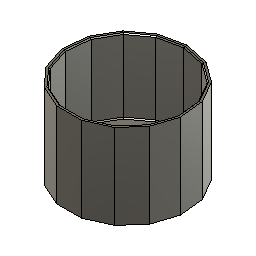
BraunBowl (Autodesk Fusion 360 design; units mm, degrees)
Autodesk Fusion 360 part; units mm, degrees
sketch "Sketch1" plane through (0, 0, 0) normal (0, 1, 0) x (1, 0, 0)
  line L0 (0, 59) -> (-23.9975, 53.8992)
  line L1 (-23.9975, 53.8992) -> (-43.8455, 39.4787)
  line L2 (-43.8455, 39.4787) -> (-56.1123, 18.232)
  line L3 (-56.1123, 18.232) -> (-58.6768, -6.1672)
  line L4 (-58.6768, -6.1672) -> (-51.0955, -29.5)
  line L5 (-51.0955, -29.5) -> (-34.6793, -47.732)
  line L6 (-34.6793, -47.732) -> (-12.2668, -57.7107)
  line L7 (-12.2668, -57.7107) -> (12.2668, -57.7107)
  line L8 (12.2668, -57.7107) -> (34.6793, -47.732)
  line L9 (34.6793, -47.732) -> (51.0955, -29.5)
  line L10 (51.0955, -29.5) -> (58.6768, -6.1672)
  line L11 (58.6768, -6.1672) -> (56.1123, 18.232)
  line L12 (56.1123, 18.232) -> (43.8455, 39.4787)
  line L13 (43.8455, 39.4787) -> (23.9975, 53.8992)
  line L14 (23.9975, 53.8992) -> (0, 59)
extrude "Extrude1" add sketch "Sketch1" along normal blind 84
sketch "Sketch2" plane through (0, 84, 0) normal (0, 1, 0) x (-1, 0, 0)
  line L0 (0, -56) -> (22.7773, -51.1585)
  line L1 (22.7773, -51.1585) -> (41.6161, -37.4713)
  line L2 (41.6161, -37.4713) -> (53.2592, -17.305)
  line L3 (53.2592, -17.305) -> (55.6932, 5.8536)
  line L4 (55.6932, 5.8536) -> (48.4974, 28)
  line L5 (48.4974, 28) -> (32.916, 45.305)
  line L6 (32.916, 45.305) -> (11.6431, 54.7763)
  line L7 (11.6431, 54.7763) -> (-11.6431, 54.7763)
  line L8 (-11.6431, 54.7763) -> (-32.916, 45.305)
  line L9 (-32.916, 45.305) -> (-48.4974, 28)
  line L10 (-48.4974, 28) -> (-55.6932, 5.8536)
  line L11 (-55.6932, 5.8536) -> (-53.2592, -17.305)
  line L12 (-53.2592, -17.305) -> (-41.6161, -37.4713)
  line L13 (-41.6161, -37.4713) -> (-22.7773, -51.1585)
  line L14 (-22.7773, -51.1585) -> (0, -56)
  line L15 (-23.9975, -53.8992) -> (0, -59)
  line L16 (0, -59) -> (23.9975, -53.8992)
  line L17 (23.9975, -53.8992) -> (43.8455, -39.4787)
  line L18 (43.8455, -39.4787) -> (56.1123, -18.232)
  line L19 (56.1123, -18.232) -> (58.6768, 6.1672)
  line L20 (58.6768, 6.1672) -> (51.0955, 29.5)
  line L21 (51.0955, 29.5) -> (34.6793, 47.732)
  line L22 (34.6793, 47.732) -> (12.2668, 57.7107)
  line L23 (12.2668, 57.7107) -> (-12.2668, 57.7107)
  line L24 (-12.2668, 57.7107) -> (-34.6793, 47.732)
  line L25 (-34.6793, 47.732) -> (-51.0955, 29.5)
  line L26 (-51.0955, 29.5) -> (-58.6768, 6.1672)
  line L27 (-58.6768, 6.1672) -> (-56.1123, -18.232)
  line L28 (-56.1123, -18.232) -> (-43.8455, -39.4787)
  line L29 (-43.8455, -39.4787) -> (-23.9975, -53.8992)
  dimension "d4" = 56
  measures "d4" distance of L0.start origin
extrude "Extrude2" cut sketch "Sketch2" against normal blind 72.8 contours L0 L1 L2 L3 L4 L5 L6 L7 L8 L9 L10 L11 L12 L13 L14
sketch "Sketch3" plane through (0, 11.2, 0) normal (0, 1, 0) x (-1, 0, 0)
  line L0 (-22.7773, -51.1585) -> (0, -56)
  line L1 (0, -56) -> (22.7773, -51.1585)
  line L2 (22.7773, -51.1585) -> (41.6161, -37.4713)
  line L3 (41.6161, -37.4713) -> (53.2592, -17.305)
  line L4 (53.2592, -17.305) -> (55.6932, 5.8536)
  line L5 (55.6932, 5.8536) -> (48.4974, 28)
  line L6 (48.4974, 28) -> (32.916, 45.305)
  line L7 (32.916, 45.305) -> (11.6431, 54.7763)
  line L8 (11.6431, 54.7763) -> (-11.6431, 54.7763)
  line L9 (-11.6431, 54.7763) -> (-32.916, 45.305)
  line L10 (-32.916, 45.305) -> (-48.4974, 28)
  line L11 (-48.4974, 28) -> (-55.6932, 5.8536)
  line L12 (-55.6932, 5.8536) -> (-53.2592, -17.305)
  line L13 (-53.2592, -17.305) -> (-41.6161, -37.4713)
  line L14 (-41.6161, -37.4713) -> (-22.7773, -51.1585)
  circle A0 centre (0, 0) radius 7.5
  dimension "d7" = 15
  constraint coincident A0.centre origin
  measures "d7" diameter of A0
extrude "Extrude3" add sketch "Sketch3" along normal blind 8 contours A0
chamfer "Chamfer1" distance 8 angle 45 1 edges at (6.9925, 11.2, 2.7121)
sketch "Sketch4" plane through (0, 19.2, 0) normal (0, 1, 0) x (-1, 0, 0)
  circle A0 centre (0, 0) radius 7.5
  circle A1 centre (0, 0) radius 3.9
  dimension "d11" = 7.8
  constraint coincident A0.centre A1.centre
  measures "d11" diameter of A1
extrude "Extrude4" cut sketch "Sketch4" against normal blind 14 contours A1
chamfer "Chamfer2" distance 1 angle 45 15 edges at (54.4762, 84, -5.7257) (47.4376, 84, -27.3881) (32.1967, 84, -44.3149) (-11.3886, 84, -53.5793) (11.3886, 84, -53.5793) (-32.1967, 84, -44.3149) (-47.4376, 84, -27.3881) (-54.4762, 84, -5.7257) (-52.0953, 84, 16.9268) (-40.7067, 84, 36.6525) (-22.2795, 84, 50.0406) (0, 84, 54.7763) (22.2795, 84, 50.0406) (40.7067, 84, 36.6525) (52.0953, 84, 16.9268)
chamfer "Chamfer4" distance 1 angle 45 3 edges at (-11.3886, 11.2, -53.5793) (11.3886, 11.2, -53.5793) (32.1967, 11.2, -44.3149) 1 faces at (-35.8936, 11.2, -21.1689)
sketch "Sketch7" plane through (0, 0, 0) normal (0, -1, 0) x (1, 0, 0)
  line L0 (0, -59) -> (23.9975, -53.8992)
  line L1 (23.9975, -53.8992) -> (43.8455, -39.4787)
  line L2 (43.8455, -39.4787) -> (56.1123, -18.232)
  line L3 (56.1123, -18.232) -> (58.6768, 6.1672)
  line L4 (58.6768, 6.1672) -> (51.0955, 29.5)
  line L5 (51.0955, 29.5) -> (34.6793, 47.732)
  line L6 (34.6793, 47.732) -> (12.2668, 57.7107)
  line L7 (12.2668, 57.7107) -> (-12.2668, 57.7107)
  line L8 (-12.2668, 57.7107) -> (-34.6793, 47.732)
  line L9 (-34.6793, 47.732) -> (-51.0955, 29.5)
  line L10 (-51.0955, 29.5) -> (-58.6768, 6.1672)
  line L11 (-58.6768, 6.1672) -> (-56.1123, -18.232)
  line L12 (-56.1123, -18.232) -> (-43.8455, -39.4787)
  line L13 (-43.8455, -39.4787) -> (-23.9975, -53.8992)
  line L14 (-23.9975, -53.8992) -> (0, -59)
  line L15 (0, -51.6115) -> (19.7509, -47.6828)
  line L16 (19.7509, -47.6828) -> (36.4949, -36.4949)
  line L17 (36.4949, -36.4949) -> (47.6828, -19.7509)
  line L18 (47.6828, -19.7509) -> (51.6115, 0)
  line L19 (51.6115, 0) -> (47.6828, 19.7509)
  line L20 (47.6828, 19.7509) -> (36.4949, 36.4949)
  line L21 (36.4949, 36.4949) -> (19.7509, 47.6828)
  line L22 (19.7509, 47.6828) -> (0, 51.6115)
  line L23 (0, 51.6115) -> (-19.7509, 47.6828)
  line L24 (-19.7509, 47.6828) -> (-36.4949, 36.4949)
  line L25 (-36.4949, 36.4949) -> (-47.6828, 19.7509)
  line L26 (-47.6828, 19.7509) -> (-51.6115, 0)
  line L27 (-51.6115, 0) -> (-47.6828, -19.7509)
  line L28 (-47.6828, -19.7509) -> (-36.4949, -36.4949)
  line L29 (-36.4949, -36.4949) -> (-19.7509, -47.6828)
  line L30 (-19.7509, -47.6828) -> (0, -51.6115)
  line L31 (-0.8802, -19.9806) -> (6.8331, -18.7965)
  line L32 (6.8331, -18.7965) -> (13.506, -14.7508)
  line L33 (13.506, -14.7508) -> (18.1228, -8.4595)
  line L34 (18.1228, -8.4595) -> (19.9806, -0.8802)
  line L35 (19.9806, -0.8802) -> (18.7965, 6.8331)
  line L36 (18.7965, 6.8331) -> (14.7508, 13.506)
  line L37 (14.7508, 13.506) -> (8.4595, 18.1228)
  line L38 (8.4595, 18.1228) -> (0.8802, 19.9806)
  line L39 (0.8802, 19.9806) -> (-6.8331, 18.7965)
  line L40 (-6.8331, 18.7965) -> (-13.506, 14.7508)
  line L41 (-13.506, 14.7508) -> (-18.1228, 8.4595)
  line L42 (-18.1228, 8.4595) -> (-19.9806, 0.8802)
  line L43 (-19.9806, 0.8802) -> (-18.7965, -6.8331)
  line L44 (-18.7965, -6.8331) -> (-14.7508, -13.506)
  line L45 (-14.7508, -13.506) -> (-8.4595, -18.1228)
  line L46 (-8.4595, -18.1228) -> (-0.8802, -19.9806)
  dimension "d29" = 20
  measures "d29" distance of L31.start origin
extrude "Extrude9" cut sketch "Sketch7" against normal blind 10 contours L15 L16 L17 L18 L19 L20 L21 L22 L23 L24 L25 L26 L27 L28 L29 L30
extrude "Extrude10" add 1 faces at (-21.5684, 10, -34.1002) along direction (0, -1, 0) blind 3
loft "Loft8" add section 1 face at (-15.045, 2.3333, 12.6537) section 2 face at (-40.2242, 2.3333, 30.9135)
loft "Loft9" add section 1 face at (-1.6909, 2.3333, 19.5859) section 2 face at (-6.5836, 4.6667, 50.302)
loft "Loft10" add section 1 face at (12.6537, 2.3333, 15.045) section 2 face at (30.9135, 2.3333, 40.2242)
loft "Loft11" add section 1 face at (19.5859, 2.3333, 1.6909) section 2 face at (50.302, 4.6667, 6.5836)
loft "Loft12" add section 1 face at (15.045, 2.3333, -12.6537) section 2 face at (40.2242, 2.3333, -30.9135)
loft "Loft13" add section 1 face at (1.6909, 4.6667, -19.5859) section 2 face at (6.5836, 4.6667, -50.302)
loft "Loft14" add section 1 face at (-12.6537, 2.3333, -15.045) section 2 face at (-30.9135, 2.3333, -40.2242)
loft "Loft15" add section 1 face at (-19.5859, 2.3333, -1.6909) section 2 face at (-50.302, 4.6667, -6.5836)
